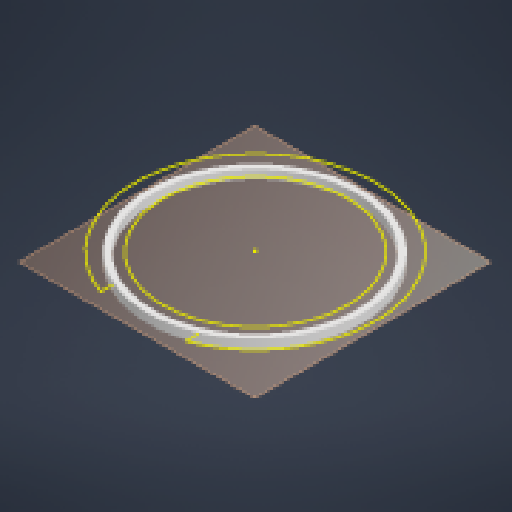
# Autodesk Inventor part: ring
Saved by Autodesk Inventor 2024 (Build 280153000, 153)
## iProperties
Created: 2023-11-07
Part Number: ring
Material: Типовые
Document SubType Name: Modeling
Designer: user
Density: 1 g/cm^3
Appearance: По умолчанию
Author: user
Autodesk Inventor part; units mm, degrees
ref_plane "YZ Plane" through (0, 0, 0) normal (1, 0, 0) x (0, 1, 0)
ref_plane "XZ Plane" through (0, 0, 0) normal (0, 1, 0) x (-1, 0, 0)
ref_plane "XY Plane" through (0, 0, 0) normal (0, 0, 1) x (1, 0, 0)
ref_plane "РабПлоскость1" through (0, 0, -3) normal (0, 0, 1) x (1, 0, 0)
sketch "Эскиз1" plane through (0, 0, -3) normal (0, 0, 1) x (1, 0, 0)
  circle A0 centre (0, 0) radius 33.125 projected
  circle A1 centre (0, 0) radius 35.125 projected
ref_plane "РабПлоскость2" through (-38, -36.68, 0) normal (0, 0, 1) x (1, 0, 0)
extrude "Выдавливание1" add sketch "Эскиз1" along normal up to surface (3 mm away)
sketch "Эскиз2" plane through (0, 0, 0) normal (0, 0, 1) x (1, 0, 0)
  circle A0 centre (0, 0) radius 30.25 projected
  arc A1 (9.9286, -36.68) -> (-9.9286, -36.68) centre (0, 0) ccw projected
  line L0 (9.9286, -36.68) -> (-9.9286, -36.68) projected
extrude "Выдавливание2" add sketch "Эскиз2" along normal blind 2
